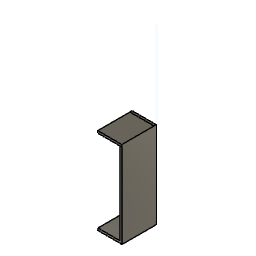
pbk (Autodesk Fusion 360 archive; units mm, degrees)
design "powerbank" references "pb2-1"
Autodesk Fusion 360 part; units mm, degrees
sketch "Sketch1" plane through (0, 0, 0) normal (0, 1, 0) x (1, 0, 0) in component "Body"
  line L0 (0, 0) -> (144, 0)
  line L1 (144, 0) -> (144, -79)
  line L2 (144, -79) -> (0, -79)
  line L3 (0, -79) -> (0, 0)
  dimension "d1" = 144
  dimension "d2" = 79
  constraint horizontal L0
  constraint vertical L1
  constraint horizontal L2
  constraint vertical L3
  constraint coincident L0.start L3.end
  measures "d1" distance of L0.start L0.end
  measures "d2" distance of L0.start L2.end
extrude "Extrude1" add sketch "Sketch1" along normal blind 2 makes body 1 in component "Body"
sketch "Sketch2" plane through (0, 0, 0) normal (0, 1, 0) x (1, 0, 0) in component "Body"
  line L0 (2, -79) -> (0, -79)
  line L1 (0, -79) -> (0, 0)
  line L2 (0, 0) -> (2, 0)
  line L3 (2, 0) -> (2, -79)
  constraint horizontal L0
  constraint vertical L1
  constraint horizontal L2
  constraint vertical L3
  constraint coincident L1.end L2.start
extrude "Extrude2" add sketch "Sketch2" along normal blind 22 bodies 1 in component "Body"
sketch "Sketch3" plane through (0, 0, 0) normal (0, 1, 0) x (1, 0, 0) in component "Body"
  line L0 (0, -79) -> (144, -79)
  line L1 (144, -79) -> (144, -77)
  line L2 (144, -77) -> (0, -77)
  line L3 (0, -77) -> (0, -79)
  constraint horizontal L0
  constraint vertical L1
  constraint horizontal L2
  constraint vertical L3
extrude "Extrude3" add sketch "Sketch3" along normal blind 22 bodies 1 in component "Body"
sketch "Sketch4" plane through (0, 0, 0) normal (0, 1, 0) x (1, 0, 0) in component "Body"
  line L0 (0, -2) -> (144, -2)
  line L1 (144, -2) -> (144, 0)
  line L2 (144, 0) -> (0, 0)
  line L3 (0, 0) -> (0, -2)
  constraint horizontal L0
  constraint vertical L1
  constraint horizontal L2
  constraint vertical L3
extrude "Extrude4" add sketch "Sketch4" along normal blind 22 bodies 1 in component "Body"
sketch "Sketch5" plane through (0, 0, 0) normal (0, 1, 0) x (1, 0, 0) in component "Body"
  line L0 (142, -79) -> (144, -79)
  line L1 (144, -79) -> (144, 0)
  line L2 (144, 0) -> (142, 0)
  line L3 (142, 0) -> (142, -79)
  constraint horizontal L0
  constraint vertical L1
  constraint horizontal L2
  constraint vertical L3
extrude "Extrude5" add sketch "Sketch5" along normal blind 22 bodies 1 in component "Body"
sketch "Sketch6" plane through (0, 0, 0) normal (1, 0, 0) x (0, 1, 0) in component "Body"
  line L0 (22, 79) -> (0, 79)
  line L1 (0, 79) -> (0, 0)
  line L2 (0, 0) -> (22, 0)
  line L3 (22, 0) -> (22, 79)
  constraint horizontal L0
  constraint vertical L1
  constraint horizontal L2
  constraint vertical L3
  constraint coincident L1.end L2.start
sketch "Sketch1 (2)" plane through (0, 0, 0) normal (0, 1, 0) x (1, 0, 0) in component "pb2-1 v3"
  line L0 (0, 0) -> (67, 0)
  line L1 (67, 0) -> (67, -26)
  line L2 (67, -26) -> (0, -26)
  line L3 (0, -26) -> (0, 0)
  dimension "d1_1" = 67
  dimension "d2_1" = 26
  constraint horizontal L0
  constraint vertical L1
  constraint horizontal L2
  constraint vertical L3
  constraint coincident L0.start L3.end
  measures "d1_1" distance of L1.end L2.end
  measures "d2_1" distance of L0.start L2.end
extrude "Extrude1'" add sketch "Sketch1 (2)" along normal blind 2 separate body makes body 2 in component "pb2-1 v3"
sketch "Sketch2 (2)" plane through (0, 0, 0) normal (0, 1, 0) x (1, 0, 0) in component "pb2-1 v3"
  circle A0 centre (4, -2) radius 1.5
  circle A1 centre (63, -2) radius 1.5
  circle A2 centre (4, -22) radius 1.5
  circle A3 centre (63, -22) radius 1.5
  dimension "d5_1" = 3
  dimension "d6_1" = 3
  dimension "d7_1" = 3
  dimension "d8_1" = 3
  measures "d5_1" diameter of A0
  measures "d6_1" diameter of A1
  measures "d7_1" diameter of A2
  measures "d8_1" diameter of A3
extrude "Extrude2'" add sketch "Sketch2 (2)" against normal blind 3 bodies 2 in component "pb2-1 v3"
sketch "Sketch3 (2)" plane through (0, 0, 0) normal (0, 1, 0) x (1, 0, 0) in component "pb2-1 v3"
  circle A0 centre (4, -22) radius 0.75
  circle A1 centre (4, -2) radius 0.75
  circle A2 centre (63, -22) radius 0.75
  circle A3 centre (63, -2) radius 0.75
  dimension "d11_1" = 1.5
  dimension "d12_1" = 1.5
  dimension "d13" = 1.5
  dimension "d14" = 1.5
  measures "d11_1" diameter of A0
  measures "d12_1" diameter of A1
  measures "d13" diameter of A2
  measures "d14" diameter of A3
extrude "Extrude3'" add sketch "Sketch3 (2)" against normal blind 7 contours A0 bodies 2 in component "pb2-1 v3"
sketch "Sketch4 (2)" plane through (0, 0, 0) normal (0, 1, 0) x (1, 0, 0) in component "pb2-1 v3"
  circle A0 centre (4, -2) radius 0.75
  dimension "d17" = 1.5
  measures "d17" diameter of A0
extrude "Extrude4'" add sketch "Sketch4 (2)" against normal blind 7 bodies 2 in component "pb2-1 v3"
sketch "Sketch5 (2)" plane through (0, 0, 0) normal (0, 1, 0) x (1, 0, 0) in component "pb2-1 v3"
  circle A0 centre (63, -22) radius 0.75
  dimension "d20" = 1.5
  measures "d20" diameter of A0
extrude "Extrude5'" add sketch "Sketch5 (2)" against normal blind 7 bodies 2 in component "pb2-1 v3"
sketch "Sketch6 (2)" plane through (0, 0, 0) normal (0, 1, 0) x (1, 0, 0) in component "pb2-1 v3"
  circle A0 centre (63, -2) radius 0.75
  dimension "d23" = 1.5
  measures "d23" diameter of A0
extrude "Extrude6" add sketch "Sketch6 (2)" against normal blind 7 bodies 2 in component "pb2-1 v3"
sketch "Sketch1 (3)" plane through (-39.2903, 0, 0) normal (-1, 0, 0) x (0, -1, 0)
sketch "Sketch2 (3)" plane through (0, 0, 0) normal (1, 0, 0) x (0, 1, 0)
sketch "Sketch3 (3)" plane through (0, 0, 0) normal (0, 0, 1) x (1, 0, 0)
extrude "Extrude7" add 1 faces at (67, 0.6667, 8.6667) along direction (1, 0, 0) blind 6 on bodies 2 bodies 2 in component "pb2-1 v3"
extrude "Extrude8" add 1 faces at (0, 0.6667, 17.3333) along direction (-1, 0, 0) blind 6 on bodies 2 bodies 2 in component "pb2-1 v3"
extrude "Extrude9" cut 1 faces at (4.125, -7, 21.7835) along direction (0, 1, 0) blind 2 on bodies 2 bodies 2 in component "pb2-1 v3"
extrude "Extrude10" cut 1 faces at (4.0832, -7, 1.788) along direction (0, 1, 0) blind 2 on bodies 2 bodies 2 in component "pb2-1 v3"
extrude "Extrude11" cut 1 faces at (62.7329, -7, 1.8045) along direction (0, 1, 0) blind 2 on bodies 2 bodies 2 in component "pb2-1 v3"
extrude "Extrude12" cut 1 faces at (63.0556, -7, 22.2437) along direction (0, 1, 0) blind 2 on bodies 2 bodies 2 in component "pb2-1 v3"
sketch "Sketch4 (3)" plane through (-39.2903, 0, 0) normal (-1, 0, 0) x (0, -1, 0)
move_body "Move1" bodies 2 to x (1, 0, 0) y (0, 1, 0) z (0, 0, 1) at (0.5, 0, 0) in component "pb2-1 v3"
sketch "Sketch5 (3)" plane through (-39.2903, 0, 0) normal (-1, 0, 0) x (0, -1, 0)
  line L0 (-15, 53) -> (-13, 53)
  line L1 (-13, 53) -> (-13, -26)
  line L2 (-13, -26) -> (-15, -26)
  line L3 (-15, -26) -> (-15, 53)
  constraint horizontal L0
  constraint vertical L1
  constraint horizontal L2
  constraint vertical L3
extrude "Extrude13" add sketch "Sketch5 (3)" against normal blind 2 sketch seen with x (0, 1, 0) y (0, 0, 1) z (1, 0, 0) at (20.5466, 39.2903, 12.1631) bodies 2 in component "pb2-1 v3"
sketch "Sketch6 (3)" plane through (0, 0, 0) normal (1, 0, 0) x (0, 1, 0)
move_body "Move2" bodies 2 to x (1, 0, 0) y (0, 1, 0) z (0, 0, 1) at (0, 13, 0) in component "pb2-1 v3"
move_body "Move3" bodies 2 to x (1, 0, 0) y (0, 1, 0) z (0, 0, 1) at (0, 1, 119) in component "pb2-1 v3"
move_body "Move4" bodies 2 to x (1, 0, 0) y (0, 1, 0) z (0, 0, 1) at (22.2499, 0, -99.9987) in component "pb2-1 v3"
move_body "Move5" bodies 2 to x (1, 0, 0) y (0, 1, 0) z (0, 0, 1) at (0, 0, -5) in component "pb2-1 v3"
move_body "Move6" bodies 2 to x (1, 0, 0) y (0, 1, 0) z (0, 0, 1) at (4, 0, 0) in component "pb2-1 v3"
move_body "Move7" bodies 2 to x (1, 0, 0) y (0, 1, 0) z (0, 0, 1) at (0, 0, -2) in component "pb2-1 v3"
move_body "Move8" bodies 2 to x (1, 0, 0) y (0, 1, 0) z (0, 0, 1) at (0, 25, 0) in component "pb2-1 v3"
sketch "Sketch7" plane through (-0.2903, 0, 0) normal (-1, 0, 0) x (0, -1, 0)
  line L0 (-25.0013, 79.2033) -> (-25.0013, 79.2499)
  line L1 (-25.0013, 79.2499) -> (-27.0013, 79.2499)
  line L2 (-27.0013, 79.2499) -> (-27.0013, 0.2499)
  line L3 (-27.0013, 0.2499) -> (-25.8382, 0.2499)
  line L4 (-25.8382, 0.2499) -> (-25.8382, 0.2033)
  line L5 (-25.8382, 0.2033) -> (0.1618, 0.2033)
  line L6 (0.1618, 0.2033) -> (0.1618, 79.2033)
  line L7 (0.1618, 79.2033) -> (-25.0013, 79.2033)
  circle A0 centre (-1.8382, 10.2033) radius 1.5
  circle A1 centre (-21.8382, 69.2033) radius 1.5
  circle A2 centre (-21.8382, 10.2033) radius 1.5
  circle A3 centre (-1.8382, 69.2033) radius 1.5
  line L8 (-27.0013, 79.2499) -> (-24.8872, 79.2499)
  line L9 (-24.8872, 79.2499) -> (-24.8872, 0.2033)
  line L10 (-24.8872, 0.2033) -> (-27.0013, 0.2033)
  line L11 (-27.0013, 0.2033) -> (-27.0013, 79.2499)
  constraint horizontal L8
  constraint vertical L9
  constraint horizontal L10
  constraint vertical L11
  constraint coincident L5 L9.end
  constraint coincident L1.end L2.start
extrude "Extrude14" add sketch "Sketch7" along normal blind 20 contours L0 L1 L2 L3 L4 L5 L7 L8 L9 L10 L11 sketch seen with x (0, 1, 0) y (0, 0, 1) z (1, 0, 0) at (20.5466, 39.2903, 12.1631) bodies 2 in component "pb2-1 v3"
sketch "Sketch8" plane through (0, -0.1618, 0) normal (0, -1, 0) x (1, 0, 0)
  line L0 (-0.2903, 79.2033) -> (-0.2903, 0.2033)
  line L1 (-0.2903, 0.2033) -> (1.7097, 0.2033)
  line L2 (1.7097, 0.2033) -> (1.7097, 79.2033)
  line L3 (1.7097, 79.2033) -> (-0.2903, 79.2033)
sketch "Sketch9" plane through (0, 0, 0) normal (0, 0, 1) x (1, 0, 0)
sketch "Sketch10" plane through (0, 0, 0) normal (0, 1, 0) x (1, 0, 0)
move_body "Move9" bodies 2 to x (1, 0, 0) y (0, 1, 0) z (0, 0, 1) at (-0.2033, 0.2903, 0.1618) in component "pb2-1 v3"
sketch "Sketch11" plane through (0, 0, 0) normal (1, 0, 0) x (0, 1, 0)
  line L0 (25, 2) -> (0, 2)
  line L1 (0, 2) -> (0, 0)
  line L2 (0, 0) -> (25, 0)
  line L3 (25, 0) -> (25, 2)
  constraint horizontal L0
  constraint vertical L1
  constraint horizontal L2
  constraint vertical L3
  constraint coincident L1.end L2.start
extrude "Extrude15" add sketch "Sketch11" against normal blind 20 sketch seen with x (0, 1, 0) y (0, 0, 1) z (1, 0, 0) at (20.5466, 39.2903, 12.1631) bodies 2 in component "pb2-1 v3"
sketch "Sketch12" plane through (0, 0, 0) normal (1, 0, 0) x (0, 1, 0)
  line L0 (25, 79) -> (0, 79)
  line L1 (0, 79) -> (0, 77)
  line L2 (0, 77) -> (25, 77)
  line L3 (25, 77) -> (25, 79)
  constraint horizontal L0
  constraint vertical L1
  constraint horizontal L2
  constraint vertical L3
extrude "Extrude16" add sketch "Sketch12" against normal blind 20 sketch seen with x (0, 1, 0) y (0, 0, 1) z (1, 0, 0) at (20.5466, 39.2903, 12.1631) bodies 2 in component "pb2-1 v3"
sketch "Sketch13" plane through (0, 0, 0) normal (0, 1, 0) x (1, 0, 0)
move_body "Move10" bodies 2 to x (1, 0, 0) y (0, 1, 0) z (0, 0, 1) at (-0.0466, -2, -27.3249) in component "pb2-1 v3"
sketch "Sketch14" plane through (0, 0, 0) normal (0, 1, 0) x (1, 0, 0)
  line L0 (-6, -66) -> (-12, -66)
  line L1 (-12, -66) -> (-12, -53)
  line L2 (-12, -53) -> (-6, -53)
  line L3 (-6, -53) -> (-6, -66)
  line L4 (-12, -49) -> (-6, -49)
  line L5 (-6, -49) -> (-6, -36)
  line L6 (-6, -36) -> (-12, -36)
  line L7 (-12, -36) -> (-12, -49)
  line L8 (-6, -12) -> (-10, -12)
  line L9 (-10, -12) -> (-10, -20)
  line L10 (-10, -20) -> (-6, -20)
  line L11 (-6, -20) -> (-6, -12)
  line L12 (-6, -24) -> (-10, -24)
  line L13 (-10, -24) -> (-10, -32)
  line L14 (-10, -32) -> (-6, -32)
  line L15 (-6, -32) -> (-6, -24)
  constraint horizontal L0
  constraint vertical L1
  constraint horizontal L2
  constraint vertical L3
  constraint horizontal L4
  constraint vertical L5
  constraint horizontal L6
  constraint vertical L7
  constraint horizontal L8
  constraint vertical L9
  constraint horizontal L10
  constraint vertical L11
  constraint horizontal L12
  constraint vertical L13
  constraint horizontal L14
  constraint vertical L15
extrude "Extrude17" cut sketch "Sketch14" against normal blind 4 sketch seen with x (0, 1, 0) y (0, 0, 1) z (1, 0, 0) at (20.5466, 39.2903, 12.1631) bodies 2 in component "pb2-1 v3"
sketch "Sketch15" plane through (0, 0, 0) normal (0, 1, 0) x (1, 0, 0)
  line L0 (0, -2) -> (-22, -2)
  line L1 (-22, -2) -> (-22, 0)
  line L2 (-22, 0) -> (0, 0)
  line L3 (0, 0) -> (0, -2)
  constraint horizontal L0
  constraint vertical L1
  constraint horizontal L2
  constraint vertical L3
extrude "Extrude18" add sketch "Sketch15" against normal blind 5 sketch seen with x (0, 1, 0) y (0, 0, 1) z (1, 0, 0) at (20.5466, 39.2903, 12.1631) bodies 2 in component "pb2-1 v3"
move_body "Move11" bodies 2 to x (1, 0, 0) y (0, 1, 0) z (0, 0, 1) at (-79.2033, -1.7097, 0.1618) in component "pb2-1 v3"
sketch "Sketch16" plane through (0, 0, 0) normal (0, 1, 0) x (1, 0, 0)
move_body "Move12" bodies 2 to x (1, 0, 0) y (0, 1, 0) z (0, 0, 1) at (0.2499, 1.7097, 27.1631) in component "pb2-1 v3"
sketch "Sketch17" plane through (0, -0.1618, 0) normal (0, -1, 0) x (1, 0, 0)
  line L0 (-22, 0) -> (0, 0)
  line L1 (0, 0) -> (0, -2)
  line L2 (0, -2) -> (-22, -2)
  line L3 (-22, -2) -> (-22, 0)
  constraint horizontal L0
  constraint vertical L1
  constraint horizontal L2
  constraint vertical L3
extrude "Extrude19" add sketch "Sketch17" against normal blind 27 sketch seen with x (0, 1, 0) y (0, 0, 1) z (1, 0, 0) at (20.5466, 39.2903, 12.1631) bodies 2 in component "pb2-1 v3"
move_body "Move13" bodies 2 to x (1, 0, 0) y (0, 1, 0) z (0, 0, 1) at (-0.0466, 0, -27.1631) in component "pb2-1 v3"
sketch "Sketch18" plane through (0, 0, 0) normal (0, 1, 0) x (1, 0, 0)
  line L0 (-5, 12) -> (-13, 12)
  line L1 (-13, 12) -> (-13, 27)
  line L2 (-13, 27) -> (-5, 27)
  line L3 (-5, 27) -> (-5, 12)
  constraint horizontal L0
  constraint vertical L1
  constraint horizontal L2
  constraint vertical L3
extrude "Extrude20" cut sketch "Sketch18" against normal blind 5 sketch seen with x (0, 1, 0) y (0, 0, 1) z (1, 0, 0) at (20.5466, 39.2903, 12.1631) bodies 2 in component "pb2-1 v3"
sketch "Sketch19" plane through (0, 0, 0) normal (1, 0, 0) x (0, 1, 0)
sketch "Sketch20" plane through (0, 0, 0) normal (0, 1, 0) x (1, 0, 0)
  line L0 (-5, 29) -> (-13, 29)
  line L1 (-13, 29) -> (-13, 44)
  line L2 (-13, 44) -> (-5, 44)
  line L3 (-5, 44) -> (-5, 29)
  constraint horizontal L0
  constraint vertical L1
  constraint horizontal L2
  constraint vertical L3
extrude "Extrude21" cut sketch "Sketch20" against normal blind 15 sketch seen with x (0, 1, 0) y (0, 0, 1) z (1, 0, 0) at (20.5466, 39.2903, 12.1631) bodies 2 in component "pb2-1 v3"
sketch "Sketch21" plane through (0, 0, 0) normal (0, 1, 0) x (1, 0, 0)
  line L0 (-11, 56) -> (-5, 56)
  line L1 (-5, 56) -> (-5, 46)
  line L2 (-5, 46) -> (-11, 46)
  line L3 (-11, 46) -> (-11, 56)
  constraint horizontal L0
  constraint vertical L1
  constraint horizontal L2
  constraint vertical L3
extrude "Extrude22" cut sketch "Sketch21" against normal blind 5 sketch seen with x (0, 1, 0) y (0, 0, 1) z (1, 0, 0) at (20.5466, 39.2903, 12.1631) bodies 2 in component "pb2-1 v3"
sketch "Sketch22" plane through (0, 0, 0) normal (0, 0, 1) x (1, 0, 0)
sketch "Sketch23" plane through (0, 0, 0) normal (0, 1, 0) x (1, 0, 0)
  line L0 (-5, 58) -> (-11, 58)
  line L1 (-11, 58) -> (-11, 68)
  line L2 (-11, 68) -> (-5, 68)
  line L3 (-5, 68) -> (-5, 58)
  constraint horizontal L0
  constraint vertical L1
  constraint horizontal L2
  constraint vertical L3
extrude "Extrude23" cut sketch "Sketch23" against normal blind 5 sketch seen with x (0, 1, 0) y (0, 0, 1) z (1, 0, 0) at (20.5466, 39.2903, 12.1631) bodies 2 in component "pb2-1 v3"
sketch "Sketch24" plane through (0, 0, 0) normal (0, 1, 0) x (1, 0, 0)
  line L0 (-10, 12) -> (-18, 12)
  line L1 (-18, 12) -> (-18, 27)
  line L2 (-18, 27) -> (-10, 27)
  line L3 (-10, 27) -> (-10, 12)
  constraint horizontal L0
  constraint vertical L1
  constraint horizontal L2
  constraint vertical L3
extrude "Extrude24" cut sketch "Sketch24" against normal blind 5 sketch seen with x (0, 1, 0) y (0, 0, 1) z (1, 0, 0) at (20.5466, 39.2903, 12.1631) bodies 2 in component "pb2-1 v3"
sketch "Sketch25" plane through (0, 0, 0) normal (0, 1, 0) x (1, 0, 0)
  line L0 (-4, 11) -> (-10, 11)
  line L1 (-10, 11) -> (-10, 28)
  line L2 (-10, 28) -> (-4, 28)
  line L3 (-4, 28) -> (-4, 11)
  constraint horizontal L0
  constraint vertical L1
  constraint horizontal L2
  constraint vertical L3
extrude "Extrude25" add sketch "Sketch25" against normal blind 2.114 sketch seen with x (0, 1, 0) y (0, 0, 1) z (1, 0, 0) at (20.5466, 39.2903, 12.1631) bodies 2 in component "pb2-1 v3"
sketch "Sketch26" plane through (0, -0.1618, 0) normal (0, -1, 0) x (1, 0, 0)
sketch "Sketch27" plane through (0, 0, 0) normal (0, 1, 0) x (1, 0, 0)
  line L0 (-10, 29) -> (-18, 29)
  line L1 (-18, 29) -> (-18, 44)
  line L2 (-18, 44) -> (-10, 44)
  line L3 (-10, 44) -> (-10, 29)
  constraint horizontal L0
  constraint vertical L1
  constraint horizontal L2
  constraint vertical L3
extrude "Extrude26" cut sketch "Sketch27" against normal blind 5 sketch seen with x (0, 1, 0) y (0, 0, 1) z (1, 0, 0) at (20.5466, 39.2903, 12.1631) bodies 2 in component "pb2-1 v3"
sketch "Sketch28" plane through (0, 0, 0) normal (0, 1, 0) x (1, 0, 0)
  line L0 (-4, 28) -> (-10, 28)
  line L1 (-10, 28) -> (-10, 45)
  line L2 (-10, 45) -> (-4, 45)
  line L3 (-4, 45) -> (-4, 28)
  constraint horizontal L0
  constraint vertical L1
  constraint horizontal L2
  constraint vertical L3
extrude "Extrude27" add sketch "Sketch28" against normal blind 2.114 sketch seen with x (0, 1, 0) y (0, 0, 1) z (1, 0, 0) at (20.5466, 39.2903, 12.1631) bodies 2 in component "pb2-1 v3"
sketch "Sketch29" plane through (0, 0, 0) normal (0, 1, 0) x (1, 0, 0)
  line L0 (-10, 46) -> (-16, 46)
  line L1 (-16, 46) -> (-16, 56)
  line L2 (-16, 56) -> (-10, 56)
  line L3 (-10, 56) -> (-10, 46)
  constraint horizontal L0
  constraint vertical L1
  constraint horizontal L2
  constraint vertical L3
extrude "Extrude28" cut sketch "Sketch29" against normal blind 3 sketch seen with x (0, 1, 0) y (0, 0, 1) z (1, 0, 0) at (20.5466, 39.2903, 12.1631) bodies 2 in component "pb2-1 v3"
sketch "Sketch30" plane through (0, 0, 0) normal (0, 1, 0) x (1, 0, 0)
  line L0 (-4, 45) -> (-10, 45)
  line L1 (-10, 45) -> (-10, 57)
  line L2 (-10, 57) -> (-4, 57)
  line L3 (-4, 57) -> (-4, 45)
  constraint horizontal L0
  constraint vertical L1
  constraint horizontal L2
  constraint vertical L3
extrude "Extrude29" add sketch "Sketch30" against normal blind 2.114 sketch seen with x (0, 1, 0) y (0, 0, 1) z (1, 0, 0) at (20.5466, 39.2903, 12.1631) bodies 2 in component "pb2-1 v3"
sketch "Sketch31" plane through (0, 0, 0) normal (1, 0, 0) x (0, 1, 0)
sketch "Sketch32" plane through (0, 0, 0) normal (0, 1, 0) x (1, 0, 0)
  line L0 (-10, 58) -> (-16, 58)
  line L1 (-16, 58) -> (-16, 68)
  line L2 (-16, 68) -> (-10, 68)
  line L3 (-10, 68) -> (-10, 58)
  constraint horizontal L0
  constraint vertical L1
  constraint horizontal L2
  constraint vertical L3
extrude "Extrude30" cut sketch "Sketch32" against normal blind 3 sketch seen with x (0, 1, 0) y (0, 0, 1) z (1, 0, 0) at (20.5466, 39.2903, 12.1631) bodies 2 in component "pb2-1 v3"
sketch "Sketch33" plane through (0, 0, 0) normal (0, 1, 0) x (1, 0, 0)
  line L0 (-4, 57) -> (-10, 57)
  line L1 (-10, 57) -> (-10, 69)
  line L2 (-10, 69) -> (-4, 69)
  line L3 (-4, 69) -> (-4, 57)
  constraint horizontal L0
  constraint vertical L1
  constraint horizontal L2
  constraint vertical L3
extrude "Extrude31" add sketch "Sketch33" against normal blind 2.114 sketch seen with x (0, 1, 0) y (0, 0, 1) z (1, 0, 0) at (20.5466, 39.2903, 12.1631) bodies 2 in component "pb2-1 v3"
extrude "Extrude32" add 1 faces at (-32.1667, 38.6236, -15) along direction (0, 0, -1) blind 4 on bodies 2 bodies 2 in component "pb2-1 v3"
extrude "Extrude33" add 1 faces at (19.8333, 31.2903, -15.1618) along direction (0, 0, -1) blind 4 on bodies 2 bodies 2 in component "pb2-1 v3"
component "Body" placed x (1, 0, 0) y (0, 1, 0) z (0, 0, 1) at (0, 0, 0)
component "Lid" placed x (1, 0, 0) y (0, 1, 0) z (0, 0, 1) at (0, 0, 0)
component "pb2-1 v3" placed x (0, 0, 1) y (1, 0, 0) z (0, 1, 0) at (-39.2903, -12.1631, -20.5466)

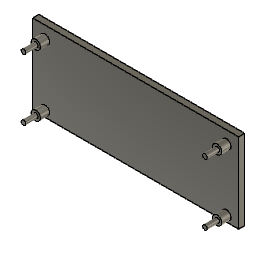
design "pb2-1"
Autodesk Fusion 360 part; units mm, degrees
sketch "Sketch1" plane through (0, 0, 0) normal (0, 1, 0) x (1, 0, 0)
  line L0 (0, 0) -> (67, 0)
  line L1 (67, 0) -> (67, -26)
  line L2 (67, -26) -> (0, -26)
  line L3 (0, -26) -> (0, 0)
  dimension "d1" = 67
  dimension "d2" = 26
  constraint horizontal L0
  constraint vertical L1
  constraint horizontal L2
  constraint vertical L3
  constraint coincident L0.start L3.end
  measures "d1" distance of L1.end L2.end
  measures "d2" distance of L0.start L2.end
extrude "Extrude1" add sketch "Sketch1" along normal blind 2
sketch "Sketch2" plane through (0, 0, 0) normal (0, 1, 0) x (1, 0, 0)
  circle A0 centre (4, -2) radius 1.5
  circle A1 centre (63, -2) radius 1.5
  circle A2 centre (4, -22) radius 1.5
  circle A3 centre (63, -22) radius 1.5
  dimension "d5" = 3
  dimension "d6" = 3
  dimension "d7" = 3
  dimension "d8" = 3
  measures "d5" diameter of A0
  measures "d6" diameter of A1
  measures "d7" diameter of A2
  measures "d8" diameter of A3
extrude "Extrude2" add sketch "Sketch2" against normal blind 3
sketch "Sketch3" plane through (0, 0, 0) normal (0, 1, 0) x (1, 0, 0)
  circle A0 centre (4, -22) radius 0.75
  circle A1 centre (4, -2) radius 0.75
  circle A2 centre (63, -22) radius 0.75
  circle A3 centre (63, -2) radius 0.75
  dimension "d11" = 1.5
  dimension "d12" = 1.5
  dimension "d13" = 1.5
  dimension "d14" = 1.5
  measures "d11" diameter of A0
  measures "d12" diameter of A1
  measures "d13" diameter of A2
  measures "d14" diameter of A3
extrude "Extrude3" add sketch "Sketch3" against normal blind 7 contours A0
sketch "Sketch4" plane through (0, 0, 0) normal (0, 1, 0) x (1, 0, 0)
  circle A0 centre (4, -2) radius 0.75
  dimension "d17" = 1.5
  measures "d17" diameter of A0
extrude "Extrude4" add sketch "Sketch4" against normal blind 7
sketch "Sketch5" plane through (0, 0, 0) normal (0, 1, 0) x (1, 0, 0)
  circle A0 centre (63, -22) radius 0.75
  dimension "d20" = 1.5
  measures "d20" diameter of A0
extrude "Extrude5" add sketch "Sketch5" against normal blind 7
sketch "Sketch6" plane through (0, 0, 0) normal (0, 1, 0) x (1, 0, 0)
  circle A0 centre (63, -2) radius 0.75
  dimension "d23" = 1.5
  measures "d23" diameter of A0
extrude "Extrude6" add sketch "Sketch6" against normal blind 7
